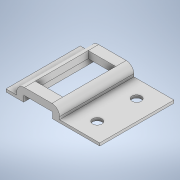
# Autodesk Inventor part: Servo Holder Cap
Saved by Autodesk Inventor 2020 (Build 240168000, 168)
## iProperties
Created: 2020-03-17
Part Number: Servo Holder Cap
Material: Generic
Document SubType Name: Modeling
Designer: varun
Density: 1 g/cm^3
Appearance: Default
Author: varun
Autodesk Inventor part; units mm, degrees
ref_plane "YZ Plane" through (0, 0, 0) normal (1, 0, 0) x (0, 1, 0)
ref_plane "XZ Plane" through (0, 0, 0) normal (0, 1, 0) x (-1, 0, 0)
ref_plane "XY Plane" through (0, 0, 0) normal (0, 0, 1) x (1, 0, 0)
sketch "Sketch1" plane through (0, 0, 0) normal (0, 0, 1) x (1, 0, 0)
  line L0 (-5.575, 0) -> (6.925, 0)
  line L1 (6.925, 2.35) -> (6.925, 0)
  line L2 (-5.575, 2.35) -> (-5.575, 0)
  line L3 (-5.275, 2.65) -> (6.625, 2.65)
  arc A0 (-5.275, 2.65) -> (-5.575, 2.35) centre (-5.275, 2.35) ccw
  arc A1 (6.925, 2.35) -> (6.625, 2.65) centre (6.625, 2.35) ccw
  line L4 (-5.575, 0) -> (6.925, 0)
  line L5 (-8.575, 0) -> (-8.575, 2.35)
  arc A2 (-5.275, 5.65) -> (-8.575, 2.35) centre (-5.275, 2.35) ccw
  line L6 (-5.275, 5.65) -> (6.625, 5.65)
  arc A3 (9.925, 2.35) -> (6.625, 5.65) centre (6.625, 2.35) ccw
  line L7 (9.925, 2.35) -> (9.925, 0)
  line L8 (-8.575, 0) -> (9.925, 0)
  line L9 (6.925, 1.175) -> (14.545, 1.175)
  line L10 (14.545, 1.175) -> (14.545, 0)
  line L11 (14.545, 0) -> (6.925, 0)
  line L12 (6.925, 1.175) -> (6.925, 0)
  line L13 (-5.575, 1.175) -> (-13.195, 1.175)
  line L14 (-5.575, 1.175) -> (2.045, 1.175) construction
  line L15 (-13.195, 1.175) -> (-13.195, 0)
  line L16 (-13.195, 0) -> (14.545, 0)
  point P0 (0, 0)
  point P1 (-8.575, 1.175)
  point P2 (-5.275, 2.65)
  point P3 (9.925, 1.175)
  dimension "d0" = 3
  dimension "d1" = 3
  dimension "d2" = 7.62
  dimension "d3" = 7.62
  dimension "d4" = 180
  constraints: 34 end point, 8 point on circle, 6 perpendicular, 4 centre point, 3 horizontal, 2 collinear, 2 midpoint, 1 point on line, 3 other
  measures "d0" distance between parallel lines of L2 L5
  measures "d1" distance between parallel lines of L3 L6
  measures "d2" distance of L9.start L9.end
  measures "d3" distance of L13.start L13.end
  measures "d4" angle of L13 L14
extrude "Extrusion1" add sketch "Sketch1" along normal blind 32.0548 contours L8 L5 L13 L2 | L1 L9 L7 L8 | L13 L5 A2 L6 A3 L7 L9 L1 A1 L3 A0 L2 | L16 L15 L13 L5 | L7 L9 L10 L11
sketch "Sketch2" plane through (-5.275, 5.65, 0) normal (0, 1, 0) x (1, 0, 0)
  line L0 (0, -32.0548) -> (11.9, -32.0548) projected
  line L1 (5.95, -32.0548) -> (5.95, -15.939)
  line L2 (0, 0) -> (0, -32.0548) projected
  line L3 (0, -4.509) -> (11.9, -4.509)
  line L4 (11.9, -4.509) -> (11.9, -27.369)
  line L5 (11.9, -27.369) -> (0, -27.369)
  line L6 (0, -27.369) -> (0, -4.509)
  line L7 (0, -4.509) -> (11.9, -27.369) construction
  line L8 (11.9, -4.509) -> (0, -27.369) construction
  line L9 (11.9, 0) -> (0, 0) projected
  dimension "d7" = 22.86
  constraints: 14 end point, 4 parallel, 3 midpoint, 1 horizontal, 1 perpendicular
  measures "d7" distance of L3.end L4.end
extrude "Extrusion2" cut sketch "Sketch2" against normal blind 32.0548 contours L2 L3 L4 L5
sketch "Sketch3" plane through (14.545, 0, 0) normal (1, 0, 0) x (0, 0, -1)
  line L0 (0, 0) -> (0, 1.175) projected
  line L1 (0, 1.175) -> (-32.0548, 1.175) projected
  line L2 (-32.0548, 0) -> (-32.0548, 1.175) projected
  line L3 (0, 0) -> (-32.0548, 0) projected
extrude "Extrusion3" add sketch "Sketch3" along normal blind 12.7
sketch "Sketch4" plane through (9.925, 1.175, 32.0548) normal (0, 1, 0) x (1, 0, 0)
  line L0 (0, 32.0548) -> (17.32, 32.0548) projected
  line L1 (0, 32.0548) -> (0, 0) projected
  line L2 (0, 0) -> (17.32, 0) projected
  line L3 (17.32, 32.0548) -> (17.32, 0) projected
  line L4 (0, 0) -> (8.7376, 0)
  line L5 (-3, 0) -> (17.32, 0) projected
  line L6 (8.7376, 0) -> (8.7376, 7.5184)
  circle A0 centre (8.7376, 7.5184) radius 2
  line L7 (0, 32.0548) -> (8.7376, 32.0548)
  line L8 (-3, 32.0548) -> (17.32, 32.0548) projected
  line L9 (8.7376, 32.0548) -> (8.7376, 24.5364)
  circle A1 centre (8.7376, 24.5364) radius 2
  point P0 (-9.925, 32.0548)
  dimension "d12" = 8.7376
  dimension "d13" = 7.5184
  dimension "d14" = 4
  dimension "d15" = 8.7376
  dimension "d16" = 7.5184
  dimension "d17" = 90
  dimension "d18" = 4
  constraints: 8 end point, 2 centre point, 2 coincident, 2 point on line, 1 parallel, 1 perpendicular
  measures "d12" distance of L1.end L4.end
  measures "d13" distance of L4.end L6.end
  measures "d14" diameter of A0
  measures "d15" distance of L0.start L7.end
  measures "d16" distance of L7.end L9.end
  measures "d17" angle of L7 L9
  measures "d18" diameter of A1
extrude "Extrusion4" cut sketch "Sketch4" against normal up to surface (1.175 mm away) contours A0 | A1
body "Solid1"
